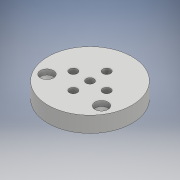
# Autodesk Inventor part: slider_wheel
Saved by Autodesk Inventor 2017 (Build 210142000, 142)
## iProperties
Created: 2018-02-07
Part Number: slider_wheel
Material: Generic
Document SubType Name: Modeling
Designer: Nic
Density: 1 g/cm^3
Appearance: Default
Author: Nic
Autodesk Inventor part; units mm, degrees
ref_plane "YZ Plane" through (0, 0, 0) normal (1, 0, 0) x (0, 1, 0)
ref_plane "XZ Plane" through (0, 0, 0) normal (0, 1, 0) x (-1, 0, 0)
ref_plane "XY Plane" through (0, 0, 0) normal (0, 0, 1) x (1, 0, 0)
sketch "Sketch1" plane through (0, 0, 0) normal (0, 0, 1) x (1, 0, 0)
  circle A0 centre (0, 0) radius 16
  dimension "d0" = 32
  constraints: 1 centre point, 1 coincident
  measures "d0" diameter of A0
extrude "Extrusion1" add sketch "Sketch1" along normal blind 6
sketch "Sketch2" plane through (0, 0, 6) normal (0, 0, 1) x (1, 0, 0)
  circle A0 centre (-10.3923, -6) radius 2.5
  circle A1 centre (10.3923, -6) radius 2.5
  circle A2 centre (0, 0) radius 12 construction
  line L0 (-10.3923, -6) -> (0, 0) construction
  line L1 (0, 0) -> (10.3923, -6) construction
  line L2 (0, 0) -> (0, 12) construction
  dimension "d3" = 120
  dimension "d4" = 5
  dimension "d5" = 24
  constraints: 6 end point, 3 centre point, 3 point on circle, 1 coincident, 1 equal radius, 1 vertical, 1 other
  measures "d3" angle of L1 L0
  measures "d4" diameter of A0
  measures "d5" diameter of A2
sketch "Sketch3" plane through (0, 0, 6) normal (0, 0, 1) x (1, 0, 0)
  circle A0 centre (0, 0) radius 1.5
  circle A1 centre (0, 6.35) radius 1.5
  circle A2 centre (0, 0) radius 6.35 construction
  circle A3 centre (-6.35, 0) radius 1.5
  circle A4 centre (0, -6.35) radius 1.5
  circle A5 centre (6.35, 0) radius 1.5
  dimension "d8" = 3
  dimension "d13" = 3
  dimension "d14" = 6.35
  dimension "d17" = 360
  constraints: 5 centre point, 2 coincident, 2 vertical alignment, 11 other
  measures "d8" diameter of A0
  measures "d13" diameter of A1
  measures "d14" distance of A1.centre point (0, 0)
extrude "Extrusion3" cut sketch "Sketch3" against normal up to next
extrude "Extrusion4" cut sketch "Sketch2" against normal blind 2
body "Solid1"
